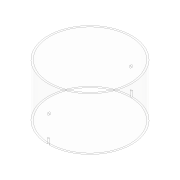
# Autodesk Inventor part: pipe_70mm
Saved by Autodesk Inventor 2018 (Build 220112000, 112)
## iProperties
Created: 2019-01-23
Part Number: pipe_70mm
Material: Generic
Document SubType Name: Modeling
Designer: Koki
Density: 1 g/cm^3
Appearance: Clear - Light
Author: Koki
Autodesk Inventor part; units mm, degrees
ref_plane "YZ Plane" through (0, 0, 0) normal (1, 0, 0) x (0, 1, 0)
ref_plane "XZ Plane" through (0, 0, 0) normal (0, 1, 0) x (-1, 0, 0)
ref_plane "XY Plane" through (0, 0, 0) normal (0, 0, 1) x (1, 0, 0)
sketch "Sketch1" plane through (0, 0, 0) normal (0, 0, 1) x (1, 0, 0)
  circle A0 centre (0, 0) radius 38.1
  circle A1 centre (0, 0) radius 39.6875
  dimension "d0" = 76.2
  dimension "d1" = 79.375
  constraints: 2 centre point, 2 coincident
  measures "d0" diameter of A0
  measures "d1" diameter of A1
extrude "Extrusion1" add sketch "Sketch1" along normal blind 50
sketch "Sketch2" plane through (0, 0, 0) normal (1, 0, 0) x (0, 1, 0)
  circle A0 centre (0, 30) radius 1
  line L0 (-39.6875, 0) -> (39.6875, 0) projected
  point P0 (0, 0)
  dimension "d4" = 2
  dimension "d5" = 30
  constraints: 1 centre point
  measures "d4" diameter of A0
  measures "d5" distance from line of L0 A0.centre
extrude "Extrusion2" [suppressed]
sketch "Sketch3" plane through (0, 0, 0) normal (0, 1, 0) x (-1, 0, 0)
  circle A0 centre (0, 25) radius 1
  line L0 (-39.6875, 0) -> (39.6875, 0) projected
  line L1 (39.6875, 50) -> (-39.6875, 50) projected
  point P0 (0, 0)
  dimension "d8" = 2
  dimension "d12" = 25
  constraints: 1 centre point
  measures "d8" diameter of A0
  measures "d12" distance from line of A0.centre L1
extrude "Extrusion3" cut sketch "Sketch3" along normal through all both and the other way through all
sketch "Sketch5" plane through (0, 0, 0) normal (0, 0, -1) x (-1, 0, 0)
  circle A0 centre (0, 39.6875) radius 1
  point P0 (0, 0)
  dimension "d20" = 2
  dimension "d21" = 39.6875
  constraints: 1 centre point
  measures "d20" diameter of A0
  measures "d21" distance of point (0, 0) A0.centre
extrude "Extrusion5" cut sketch "Sketch5" against normal blind 5
pattern_circular "Circular Pattern2" count 2 over 360 about axis through (0, 0, 0) along (0, 0, 1) of "Extrusion5"
body "Solid1"
